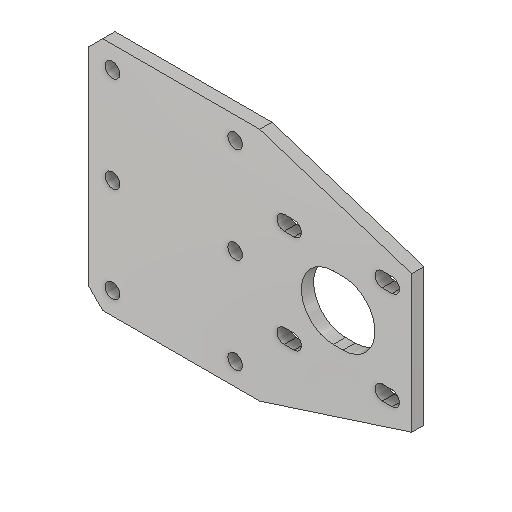
# Autodesk Inventor part: LC_ALU_3mm_X_axis_belt_idler_mount_plate
Saved by Autodesk Inventor 2026.1 (Build 301233000, 233)
## iProperties
Created: 2018-07-10
Part Number: LC_ALU_3mm_X_axis_belt_idler_mount_plate
Material: Aluminum 6061-AHC
Document SubType Name: Modeling
Designer: Andrzej
Density: 2.7 g/cm^3
Appearance: Aluminum - Polished
Author: Andrzej
Autodesk Inventor part; units mm, degrees
ref_plane "YZ Plane" through (0, 0, 0) normal (1, 0, 0) x (0, 1, 0)
ref_plane "XZ Plane" through (0, 0, 0) normal (0, 1, 0) x (-1, 0, 0)
ref_plane "XY Plane" through (0, 0, 0) normal (0, 0, 1) x (1, 0, 0)
sketch "Sketch1" plane through (0, 0, 0) normal (0, 0, 1) x (1, 0, 0)
  line L0 (-12.273, 14.9908) -> (-12.273, -33.0092)
  line L1 (-12.273, -33.0092) -> (22.727, -33.0092)
  line L2 (53.727, -23.0092) -> (53.727, 4.9908)
  line L3 (-12.273, 14.9908) -> (22.727, 14.9908)
  line L4 (22.727, 14.9908) -> (22.727, 4.9908)
  line L5 (22.727, 4.9908) -> (53.727, 4.9908)
  line L6 (22.727, 4.9908) -> (22.727, -33.0092)
  line L7 (53.727, -23.0092) -> (22.727, -23.0092)
  line L8 (22.727, -33.0092) -> (53.727, -23.0092)
  line L9 (53.727, 4.9908) -> (22.727, 14.9908)
  line L10 (29.727, 0.9908) -> (27.727, 0.9908) construction
  line L11 (29.727, 2.4908) -> (27.727, 2.4908)
  line L12 (27.727, -0.5092) -> (29.727, -0.5092)
  arc A0 (29.727, -0.5092) -> (29.727, 2.4908) centre (29.727, 0.9908) ccw
  arc A1 (27.727, 2.4908) -> (27.727, -0.5092) centre (27.727, 0.9908) ccw
  line L13 (49.727, 0.9908) -> (47.727, 0.9908) construction
  line L14 (49.727, 2.4908) -> (47.727, 2.4908)
  line L15 (47.727, -0.5092) -> (49.727, -0.5092)
  arc A2 (49.727, -0.5092) -> (49.727, 2.4908) centre (49.727, 0.9908) ccw
  arc A3 (47.727, 2.4908) -> (47.727, -0.5092) centre (47.727, 0.9908) ccw
  line L16 (29.727, -19.0092) -> (27.727, -19.0092) construction
  line L17 (29.727, -17.5092) -> (27.727, -17.5092)
  line L18 (27.727, -20.5092) -> (29.727, -20.5092)
  arc A4 (29.727, -20.5092) -> (29.727, -17.5092) centre (29.727, -19.0092) ccw
  arc A5 (27.727, -17.5092) -> (27.727, -20.5092) centre (27.727, -19.0092) ccw
  line L19 (49.727, -19.0092) -> (47.727, -19.0092) construction
  line L20 (49.727, -17.5092) -> (47.727, -17.5092)
  line L21 (47.727, -20.5092) -> (49.727, -20.5092)
  arc A6 (49.727, -20.5092) -> (49.727, -17.5092) centre (49.727, -19.0092) ccw
  arc A7 (47.727, -17.5092) -> (47.727, -20.5092) centre (47.727, -19.0092) ccw
  line L22 (39.727, -9.0092) -> (37.727, -9.0092) construction
  line L23 (39.727, -2.5092) -> (37.727, -2.5092)
  line L24 (37.727, -15.5092) -> (39.727, -15.5092)
  arc A8 (39.727, -15.5092) -> (39.727, -2.5092) centre (39.727, -9.0092) ccw
  arc A9 (37.727, -2.5092) -> (37.727, -15.5092) centre (37.727, -9.0092) ccw
  point P0 (0, 0)
  point P1 (-7.273, 10.4908)
  point P2 (-7.273, -9.0092)
  point P3 (-7.273, -28.5092)
  point P4 (17.727, 10.4908)
  point P5 (17.727, -9.0092)
  point P6 (17.727, -28.5092)
  point P7 (28.727, 0.9908)
  point P8 (48.727, 0.9908)
  point P9 (28.727, -19.0092)
  point P10 (48.727, -19.0092)
  point P11 (38.727, -9.0092)
  dimension "d0" = 48
  dimension "d2" = 28
  dimension "d3" = 35
  dimension "d4" = 5
  dimension "d5" = 5
  dimension "d6" = 4.5
  dimension "d7" = 4.5
  dimension "d8" = 24
  dimension "d9" = 20
  dimension "d10" = 20
  dimension "d13" = 10
  dimension "d14" = 10
  dimension "d44" = 4
  dimension "d45" = 66
  dimension "d46" = 4
  dimension "d47" = 10
  dimension "d53" = 31
  dimension "d54" = 2
  dimension "d55" = 3
  dimension "d56" = 2
  dimension "d57" = 3
  dimension "d58" = 2
  dimension "d59" = 3
  dimension "d60" = 2
  dimension "d61" = 3
  dimension "d62" = 2
  dimension "d63" = 13
  constraints: 60 end point, 20 point on circle, 20 tangent, 10 centre point, 6 parallel, 6 vertical alignment, 5 horizontal alignment, 5 midpoint, 5 perpendicular, 3 horizontal, 3 point on line, 2 vertical
  measures "d0" distance of L0.start L0.end
  measures "d2" distance of L2.start L2.end
  measures "d3" distance of L0.start L3.end
  measures "d4" distance from line of L0 point (-7.273, 10.491)
  measures "d5" distance from line of L4 point (17.727, 10.491)
  measures "d6" distance from line of L3 point (-7.273, 10.491)
  measures "d7" distance from line of L1 point (-7.273, -28.509)
  measures "d8" distance from line of L3 point (-7.273, -9.009)
  measures "d9" distance of L16.start L10.start
  measures "d10" distance of L10.start L13.start
  measures "d13" horizontal distance of L10.start L22.start
  measures "d14" horizontal distance of L16.start L22.start
  measures "d44" distance from line of L2 L19.start
  measures "d45" distance between parallel lines of L0 L2
  measures "d46" distance from line of L7 L19.start
  measures "d47" distance between parallel lines of L1 L7
  measures "d53" distance of L4.end L2.end
  measures "d54" distance of L10.start L10.end
  measures "d55" diameter of A1
  measures "d56" distance of L13.start L13.end
  measures "d57" diameter of A3
  measures "d58" distance of L16.start L16.end
  measures "d59" diameter of A5
  measures "d60" distance of L19.start L19.end
  measures "d61" diameter of A7
  measures "d62" distance of L22.start L22.end
  measures "d63" diameter of A9
extrude "Extrusion1" add sketch "Sketch1" along normal blind 2.5
hole "Hole1" at (-7.273, 10.4908, 0) at (-7.273, -9.0092, 0) at (-7.273, -28.5092, 0) at (17.727, 10.4908, 0) at (17.727, -9.0092, 0) at (17.727, -28.5092, 0) direction (0, 0, 1) diameter 3 end through all
chamfer "Chamfer3" distance 3 angle 45 2 edges at (-12.273, -33.0092, 1.25) (-12.273, 14.9908, 1.25)
equation "\"d5\" = d4"
equation "\"d10\" = d9"
equation "\"d13\" = 0.5 * d9"
equation "\"d14\" = d13"
equation "\"d44\" = d46"
equation "\"d46\" = -0.5 * d9 + 0.5 * d2"
equation "\"d47\" = -0.5 * d2 + 0.5 * d0"
body "Solid1"
